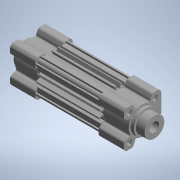
# Autodesk Inventor part: CP96S32-50(0)_BODY
Saved by Autodesk Inventor 2021 (Build 250183000, 183)
## iProperties
Part Number: CP96S32-50(0)_BODY
Material: Generic
Catalog Web Link: www.cadenas.de
Description: CP96 BODY-ISO Cylinder:Standard Double Acting,Single/Double Rod
Vendor: SMC
Document SubType Name: Modeling
Designer: partserver
Manufacturer: SMC
Mass: 188.486 g
Surface Area: 568.726 cm^2
Volume: 188.486 cm^3
Density: 1 g/cm^3
Appearance: PSOLRGB-192-192-192
Category: PARTsolutions
Company: SMC
PSOL_IDENT_0: {$CADENAS_DATA\23d-libs\smc_jp\actuator\standard_air_cylinder\cp96_c96\cp96\parts\cp96_body.prj},199
PSOL_IDENT_1: {VTYP=3D},{NB=CP96S32-50(0)_BODY},{LINA=CP96S32-50_BODY},{NN=CP96 BODY},{DATE=05.07.2021 01:48:16},
PSOL_IDENT_2: {GEOMDATE=28.11.2018 06:56:23},{VERSION=},{LINEID=10},{WBVAR=STROKE,ROD,THREAD},{WBNUMERIC=STROKE}
PSOL_IDENT_3: {NB=CP96S32-50(0)_BODY},{LINA=CP96S32-50_BODY},{KT=DUMMY},{BORE=32},{STROKE=50},{ROD=},{THREAD=0},{O
PSOL_IDENT_4: RDER=CP96S32-50},{A=22},{B=30},{D=12},{EE=G 1/8},{EEE=NPT 1/8},{EEND=9.728},{EED=9},{PL=13.0},{RT=M6
PSOL_IDENT_5: x1},{RTRA=6},{RTRP=1.00},{L12=6.0},{KK=M10x1.25},{SW=10},{G=32.0},{BG=16},{L8=94},{VD=4},{VA=4},{WA=
PSOL_IDENT_6: 4.0},{WB=7.0},{WH=26},{ZZ=146},{ZY=190},{E=47},{R=32.5},{L2=15},{L9=4},{H=48},{LC1=4.5},{LC2=25.5},{
PSOL_IDENT_7: RC1=1.5},{RC2=3.0},{RC3=6.8},{RC4=8.2},{RC5=3.9},{DC1=35.0},{DC2=36.0},{DC4=25.0},{HC=6.0},{C1=46.0}
PSOL_IDENT_8: ,{C2=42.0},{C3=30.5},{C4=34.5},{C5=16.5},{C6=20.5},{C7=17.8},{C9=17.5},{FONT=5},{SIZE=10}
NB: CP96S32-50(0)_BODY
NN: CP96 BODY
NT: ISO Cylinder:Standard Double Acting,Single/Double Rod
NBSYN: $ORDER.($THREAD.)_BODY
LINA: CP96S32-50_BODY
CATALOG: SMC (JP
BORE: 32
STROKE: 50
ROD: (-) Single rod
THREAD: on
A: 22
B: 30
D: 12
EE: G 1/8
EEE: NPT 1/8
PL: 13
RT: M6x1
L12: 6
KK: M10x1.25
SW: 10
G: 32
BG: 16
L8: 94
VD: 4
VA: 4
WA: 4
WB: 7
WH: 26
ZZ: 146
ZY: 190
E: 47
R: 32.5
L2: 15
L9: 4
H: 48
SUPPLIER: SMC
ARTICLENO: CP96S32-50(0)_BODY
BOMINFO: CP96S32-50_BODY
CREATOR: CADENAS GmbH
Title: CP96S32-50_BODY
Author: Cadenas PARTsolutions
Comments: ISO Cylinder:Standard Double Acting,Single/Double Rod
Autodesk Inventor part; units mm, degrees
sketch "Sketch_5" plane through (0, 0, 0) normal (1, 0, 0) x (0, 1, 0)
  line L0 (19.2462, 23.5) -> (14.2154, 23.5)
  arc A0 (14.2154, 23.5) -> (11.5708, 21.9163) centre (14.2154, 20.5) ccw
  line L1 (11.5708, 21.9163) -> (10.2555, 19.4602)
  arc A1 (10.2555, 19.4602) -> (9.4976, 17.0528) centre (16.25, 16.25) ccw
  arc A2 (7.3758, 15.8697) -> (9.4976, 17.0528) centre (8.0081, 17.2299) ccw
  arc A3 (7.3758, 15.8697) -> (-7.3758, 15.8697) centre (0, 0) ccw
  arc A4 (-9.4976, 17.0528) -> (-7.3758, 15.8697) centre (-8.0081, 17.2299) ccw
  arc A5 (-9.4976, 17.0528) -> (-10.2555, 19.4602) centre (-16.25, 16.25) ccw
  line L2 (-10.2555, 19.4602) -> (-11.5708, 21.9163)
  arc A6 (-11.5708, 21.9163) -> (-14.2154, 23.5) centre (-14.2154, 20.5) ccw
  line L3 (-14.2154, 23.5) -> (-19.2462, 23.5)
  arc A7 (-19.2462, 23.5) -> (-20.9749, 22.9519) centre (-19.2462, 20.5) ccw
  arc A8 (-20.9749, 22.9519) -> (-22.9519, 20.9749) centre (-16.25, 16.25) ccw
  arc A9 (-22.9519, 20.9749) -> (-23.5, 19.2462) centre (-20.5, 19.2462) ccw
  line L4 (-23.5, 19.2462) -> (-23.5, 14.2154)
  arc A10 (-23.5, 14.2154) -> (-21.9163, 11.5708) centre (-20.5, 14.2154) ccw
  line L5 (-21.9163, 11.5708) -> (-19.4602, 10.2555)
  arc A11 (-19.4602, 10.2555) -> (-17.0528, 9.4976) centre (-16.25, 16.25) ccw
  arc A12 (-15.8697, 7.3758) -> (-17.0528, 9.4976) centre (-17.2299, 8.0081) ccw
  arc A13 (-15.8697, 7.3758) -> (-15.8697, -7.3758) centre (0, 0) ccw
  arc A14 (-17.0528, -9.4976) -> (-15.8697, -7.3758) centre (-17.2299, -8.0081) ccw
  arc A15 (-17.0528, -9.4976) -> (-19.4602, -10.2555) centre (-16.25, -16.25) ccw
  line L6 (-19.4602, -10.2555) -> (-21.9163, -11.5708)
  arc A16 (-21.9163, -11.5708) -> (-23.5, -14.2154) centre (-20.5, -14.2154) ccw
  line L7 (-23.5, -14.2154) -> (-23.5, -19.2462)
  arc A17 (-23.5, -19.2462) -> (-22.9519, -20.9749) centre (-20.5, -19.2462) ccw
  arc A18 (-22.9519, -20.9749) -> (-20.9749, -22.9519) centre (-16.25, -16.25) ccw
  arc A19 (-20.9749, -22.9519) -> (-19.2462, -23.5) centre (-19.2462, -20.5) ccw
  line L8 (-19.2462, -23.5) -> (-14.2154, -23.5)
  arc A20 (-14.2154, -23.5) -> (-11.5708, -21.9163) centre (-14.2154, -20.5) ccw
  line L9 (-11.5708, -21.9163) -> (-10.2555, -19.4602)
  arc A21 (-10.2555, -19.4602) -> (-9.4976, -17.0528) centre (-16.25, -16.25) ccw
  arc A22 (-7.3758, -15.8697) -> (-9.4976, -17.0528) centre (-8.0081, -17.2299) ccw
  arc A23 (-7.3758, -15.8697) -> (7.3758, -15.8697) centre (0, 0) ccw
  arc A24 (9.4976, -17.0528) -> (7.3758, -15.8697) centre (8.0081, -17.2299) ccw
  arc A25 (9.4976, -17.0528) -> (10.2555, -19.4602) centre (16.25, -16.25) ccw
  line L10 (10.2555, -19.4602) -> (11.5708, -21.9163)
  arc A26 (11.5708, -21.9163) -> (14.2154, -23.5) centre (14.2154, -20.5) ccw
  line L11 (14.2154, -23.5) -> (19.2462, -23.5)
  arc A27 (19.2462, -23.5) -> (20.9749, -22.9519) centre (19.2462, -20.5) ccw
  arc A28 (20.9749, -22.9519) -> (22.9519, -20.9749) centre (16.25, -16.25) ccw
  arc A29 (22.9519, -20.9749) -> (23.5, -19.2462) centre (20.5, -19.2462) ccw
  line L12 (23.5, -19.2462) -> (23.5, -14.2154)
  arc A30 (23.5, -14.2154) -> (21.9163, -11.5708) centre (20.5, -14.2154) ccw
  line L13 (21.9163, -11.5708) -> (19.4602, -10.2555)
  arc A31 (19.4602, -10.2555) -> (17.0528, -9.4976) centre (16.25, -16.25) ccw
  arc A32 (15.8697, -7.3758) -> (17.0528, -9.4976) centre (17.2299, -8.0081) ccw
  arc A33 (15.8697, -7.3758) -> (15.8697, 7.3758) centre (0, 0) ccw
  arc A34 (17.0528, 9.4976) -> (15.8697, 7.3758) centre (17.2299, 8.0081) ccw
  arc A35 (17.0528, 9.4976) -> (19.4602, 10.2555) centre (16.25, 16.25) ccw
  line L14 (19.4602, 10.2555) -> (21.9163, 11.5708)
  arc A36 (21.9163, 11.5708) -> (23.5, 14.2154) centre (20.5, 14.2154) ccw
  line L15 (23.5, 14.2154) -> (23.5, 19.2462)
  arc A37 (23.5, 19.2462) -> (22.9519, 20.9749) centre (20.5, 19.2462) ccw
  arc A38 (22.9519, 20.9749) -> (20.9749, 22.9519) centre (16.25, 16.25) ccw
  arc A39 (20.9749, 22.9519) -> (19.2462, 23.5) centre (19.2462, 20.5) ccw
  constraints: 80 point on circle, 40 centre point, 32 end point
extrude "Extrusion1" add sketch "Sketch_5" along normal blind 32
sketch "Sketch_29" plane through (32, 0, 0) normal (1, 0, 0) x (0, 0, -1)
  line L0 (-23.0894, 1.6246) -> (-17.5, -0.031)
  arc A0 (-17.5, -0.031) -> (-17.3057, -2.6003) centre (0, 0) ccw
  line L1 (-17.3057, -2.6003) -> (-22.1807, -4.4229)
  line L2 (-22.1807, -4.4229) -> (-21.4365, -6.4134)
  line L3 (-21.4365, -6.4134) -> (-20.5984, -6.1)
  arc A1 (-19.5478, -8.91) -> (-20.5984, -6.1) centre (-18.6632, -6.9779) ccw
  line L4 (-19.5478, -8.91) -> (-21, -9.453)
  line L5 (-21, -9.453) -> (-21, -15.25)
  line L6 (-21, -15.25) -> (-23, -15.25)
  line L7 (-23, -15.25) -> (-23, -17.25)
  line L8 (-23, -17.25) -> (-21, -17.25)
  arc A2 (-21, -17.25) -> (-17.25, -21) centre (-17.25, -17.25) ccw
  line L9 (-17.25, -21) -> (-17.25, -23)
  line L10 (-17.25, -23) -> (-15.25, -23)
  line L11 (-15.25, -23) -> (-15.25, -21)
  line L12 (-15.25, -21) -> (-8.9843, -21)
  line L13 (-8.9843, -21) -> (-8.5904, -19.6702)
  line L14 (-8.5904, -19.6702) -> (-9.2136, -19.4856)
  line L15 (-9.2136, -19.4856) -> (-8.2196, -16.1297)
  line L16 (-8.2196, -16.1297) -> (-1.8914, -18.0042)
  line L17 (-1.8914, -18.0042) -> (-2.8854, -21.3601)
  line L18 (-2.8854, -21.3601) -> (-3.5087, -21.1755)
  line L19 (-3.5087, -21.1755) -> (-3.8779, -22.422)
  line L20 (-3.8779, -22.422) -> (-1.6246, -23.0894)
  line L21 (-1.6246, -23.0894) -> (0.031, -17.5)
  arc A3 (0.031, -17.5) -> (2.6003, -17.3057) centre (0, 0) ccw
  line L22 (2.6003, -17.3057) -> (4.4229, -22.1807)
  line L23 (4.4229, -22.1807) -> (6.4134, -21.4365)
  line L24 (6.4134, -21.4365) -> (6.1, -20.5984)
  arc A4 (8.91, -19.5478) -> (6.1, -20.5984) centre (6.9779, -18.6632) ccw
  line L25 (8.91, -19.5478) -> (9.453, -21)
  line L26 (9.453, -21) -> (15.25, -21)
  line L27 (15.25, -21) -> (15.25, -23)
  line L28 (15.25, -23) -> (17.25, -23)
  line L29 (17.25, -23) -> (17.25, -21)
  arc A5 (17.25, -21) -> (21, -17.25) centre (17.25, -17.25) ccw
  line L30 (21, -17.25) -> (23, -17.25)
  line L31 (23, -17.25) -> (23, -15.25)
  line L32 (23, -15.25) -> (21, -15.25)
  line L33 (21, -15.25) -> (21, -8.9843)
  line L34 (21, -8.9843) -> (19.6702, -8.5904)
  line L35 (19.6702, -8.5904) -> (19.4856, -9.2136)
  line L36 (19.4856, -9.2136) -> (16.1297, -8.2196)
  line L37 (16.1297, -8.2196) -> (18.0042, -1.8914)
  line L38 (18.0042, -1.8914) -> (21.3601, -2.8854)
  line L39 (21.3601, -2.8854) -> (21.1755, -3.5087)
  line L40 (21.1755, -3.5087) -> (22.422, -3.8779)
  line L41 (22.422, -3.8779) -> (23.0894, -1.6246)
  line L42 (23.0894, -1.6246) -> (17.5, 0.031)
  arc A6 (17.5, 0.031) -> (17.3057, 2.6003) centre (0, 0) ccw
  line L43 (17.3057, 2.6003) -> (22.1807, 4.4229)
  line L44 (22.1807, 4.4229) -> (21.4365, 6.4134)
  line L45 (21.4365, 6.4134) -> (20.5984, 6.1)
  arc A7 (19.5478, 8.91) -> (20.5984, 6.1) centre (18.6632, 6.9779) ccw
  line L46 (19.5478, 8.91) -> (21, 9.453)
  line L47 (21, 9.453) -> (21, 15.25)
  line L48 (21, 15.25) -> (23, 15.25)
  line L49 (23, 15.25) -> (23, 17.25)
  line L50 (23, 17.25) -> (21, 17.25)
  arc A8 (21, 17.25) -> (17.25, 21) centre (17.25, 17.25) ccw
  line L51 (17.25, 21) -> (17.25, 23)
  line L52 (17.25, 23) -> (15.25, 23)
  line L53 (15.25, 23) -> (15.25, 21)
  line L54 (15.25, 21) -> (8.9843, 21)
  line L55 (8.9843, 21) -> (8.5904, 19.6702)
  line L56 (8.5904, 19.6702) -> (9.2136, 19.4856)
  line L57 (9.2136, 19.4856) -> (8.2196, 16.1297)
  line L58 (8.2196, 16.1297) -> (1.8914, 18.0042)
  line L59 (1.8914, 18.0042) -> (2.8854, 21.3601)
  line L60 (2.8854, 21.3601) -> (3.5087, 21.1755)
  line L61 (3.5087, 21.1755) -> (3.8779, 22.422)
  line L62 (3.8779, 22.422) -> (1.6246, 23.0894)
  line L63 (1.6246, 23.0894) -> (-0.031, 17.5)
  arc A9 (-0.031, 17.5) -> (-2.6003, 17.3057) centre (0, 0) ccw
  line L64 (-2.6003, 17.3057) -> (-4.4229, 22.1807)
  line L65 (-4.4229, 22.1807) -> (-6.4134, 21.4365)
  line L66 (-6.4134, 21.4365) -> (-6.1, 20.5984)
  arc A10 (-8.91, 19.5478) -> (-6.1, 20.5984) centre (-6.9779, 18.6632) ccw
  line L67 (-8.91, 19.5478) -> (-9.453, 21)
  line L68 (-9.453, 21) -> (-15.25, 21)
  line L69 (-15.25, 21) -> (-15.25, 23)
  line L70 (-15.25, 23) -> (-17.25, 23)
  line L71 (-17.25, 23) -> (-17.25, 21)
  arc A11 (-17.25, 21) -> (-21, 17.25) centre (-17.25, 17.25) ccw
  line L72 (-21, 17.25) -> (-23, 17.25)
  line L73 (-23, 17.25) -> (-23, 15.25)
  line L74 (-23, 15.25) -> (-21, 15.25)
  line L75 (-21, 15.25) -> (-21, 8.9843)
  line L76 (-21, 8.9843) -> (-19.6702, 8.5904)
  line L77 (-19.6702, 8.5904) -> (-19.4856, 9.2136)
  line L78 (-19.4856, 9.2136) -> (-16.1297, 8.2196)
  line L79 (-16.1297, 8.2196) -> (-18.0042, 1.8914)
  line L80 (-18.0042, 1.8914) -> (-21.3601, 2.8854)
  line L81 (-21.3601, 2.8854) -> (-21.1755, 3.5087)
  line L82 (-21.1755, 3.5087) -> (-22.422, 3.8779)
  line L83 (-22.422, 3.8779) -> (-23.0894, 1.6246)
  constraints: 168 end point, 24 point on circle, 12 centre point
extrude "Extrusion2" add sketch "Sketch_29" along normal blind 80
sketch "Sketch_36" plane through (0, 23.5, 0) normal (0, 1, 0) x (1, 0, 0)
  line L0 (0, -4.5) -> (18, -4.5)
  arc A0 (18, -4.5) -> (21.5, -1) centre (18, -1) ccw
  arc A1 (22.5, 0) -> (21.5, -1) centre (22.5, -1) ccw
  line L1 (22.5, 0) -> (32, 0)
  line L2 (32, 0) -> (32, 16.25)
  line L3 (32, 16.25) -> (0, 16.25)
  line L4 (0, 16.25) -> (0, -4.5)
  constraints: 10 end point, 4 point on circle, 2 centre point
extrude "Extrusion3" add sketch "Sketch_36" against normal blind 12.25
sketch "Sketch_35" plane through (144, 0, 0) normal (1, 0, 0) x (0, 0, -1)
  line L0 (-23.5, 19.2462) -> (-23.5, 14.2154)
  arc A0 (-23.5, 14.2154) -> (-21.9163, 11.5708) centre (-20.5, 14.2154) ccw
  line L1 (-21.9163, 11.5708) -> (-19.4602, 10.2555)
  arc A1 (-19.4602, 10.2555) -> (-17.0528, 9.4976) centre (-16.25, 16.25) ccw
  arc A2 (-15.8697, 7.3758) -> (-17.0528, 9.4976) centre (-17.2299, 8.0081) ccw
  arc A3 (-15.8697, 7.3758) -> (-15.8697, -7.3758) centre (0, 0) ccw
  arc A4 (-17.0528, -9.4976) -> (-15.8697, -7.3758) centre (-17.2299, -8.0081) ccw
  arc A5 (-17.0528, -9.4976) -> (-19.4602, -10.2555) centre (-16.25, -16.25) ccw
  line L2 (-19.4602, -10.2555) -> (-21.9163, -11.5708)
  arc A6 (-21.9163, -11.5708) -> (-23.5, -14.2154) centre (-20.5, -14.2154) ccw
  line L3 (-23.5, -14.2154) -> (-23.5, -19.2462)
  arc A7 (-23.5, -19.2462) -> (-22.9519, -20.9749) centre (-20.5, -19.2462) ccw
  arc A8 (-22.9519, -20.9749) -> (-20.9749, -22.9519) centre (-16.25, -16.25) ccw
  arc A9 (-20.9749, -22.9519) -> (-19.2462, -23.5) centre (-19.2462, -20.5) ccw
  line L4 (-19.2462, -23.5) -> (-14.2154, -23.5)
  arc A10 (-14.2154, -23.5) -> (-11.5708, -21.9163) centre (-14.2154, -20.5) ccw
  line L5 (-11.5708, -21.9163) -> (-10.2555, -19.4602)
  arc A11 (-10.2555, -19.4602) -> (-9.4976, -17.0528) centre (-16.25, -16.25) ccw
  arc A12 (-7.3758, -15.8697) -> (-9.4976, -17.0528) centre (-8.0081, -17.2299) ccw
  arc A13 (-7.3758, -15.8697) -> (7.3758, -15.8697) centre (0, 0) ccw
  arc A14 (9.4976, -17.0528) -> (7.3758, -15.8697) centre (8.0081, -17.2299) ccw
  arc A15 (9.4976, -17.0528) -> (10.2555, -19.4602) centre (16.25, -16.25) ccw
  line L6 (10.2555, -19.4602) -> (11.5708, -21.9163)
  arc A16 (11.5708, -21.9163) -> (14.2154, -23.5) centre (14.2154, -20.5) ccw
  line L7 (14.2154, -23.5) -> (19.2462, -23.5)
  arc A17 (19.2462, -23.5) -> (20.9749, -22.9519) centre (19.2462, -20.5) ccw
  arc A18 (20.9749, -22.9519) -> (22.9519, -20.9749) centre (16.25, -16.25) ccw
  arc A19 (22.9519, -20.9749) -> (23.5, -19.2462) centre (20.5, -19.2462) ccw
  line L8 (23.5, -19.2462) -> (23.5, -14.2154)
  arc A20 (23.5, -14.2154) -> (21.9163, -11.5708) centre (20.5, -14.2154) ccw
  line L9 (21.9163, -11.5708) -> (19.4602, -10.2555)
  arc A21 (19.4602, -10.2555) -> (17.0528, -9.4976) centre (16.25, -16.25) ccw
  arc A22 (15.8697, -7.3758) -> (17.0528, -9.4976) centre (17.2299, -8.0081) ccw
  arc A23 (15.8697, -7.3758) -> (15.8697, 7.3758) centre (0, 0) ccw
  arc A24 (17.0528, 9.4976) -> (15.8697, 7.3758) centre (17.2299, 8.0081) ccw
  arc A25 (17.0528, 9.4976) -> (19.4602, 10.2555) centre (16.25, 16.25) ccw
  line L10 (19.4602, 10.2555) -> (21.9163, 11.5708)
  arc A26 (21.9163, 11.5708) -> (23.5, 14.2154) centre (20.5, 14.2154) ccw
  line L11 (23.5, 14.2154) -> (23.5, 19.2462)
  arc A27 (23.5, 19.2462) -> (22.9519, 20.9749) centre (20.5, 19.2462) ccw
  arc A28 (22.9519, 20.9749) -> (20.9749, 22.9519) centre (16.25, 16.25) ccw
  arc A29 (20.9749, 22.9519) -> (19.2462, 23.5) centre (19.2462, 20.5) ccw
  line L12 (19.2462, 23.5) -> (14.2154, 23.5)
  arc A30 (14.2154, 23.5) -> (11.5708, 21.9163) centre (14.2154, 20.5) ccw
  line L13 (11.5708, 21.9163) -> (10.2555, 19.4602)
  arc A31 (10.2555, 19.4602) -> (9.4976, 17.0528) centre (16.25, 16.25) ccw
  arc A32 (7.3758, 15.8697) -> (9.4976, 17.0528) centre (8.0081, 17.2299) ccw
  arc A33 (7.3758, 15.8697) -> (-7.3758, 15.8697) centre (0, 0) ccw
  arc A34 (-9.4976, 17.0528) -> (-7.3758, 15.8697) centre (-8.0081, 17.2299) ccw
  arc A35 (-9.4976, 17.0528) -> (-10.2555, 19.4602) centre (-16.25, 16.25) ccw
  line L14 (-10.2555, 19.4602) -> (-11.5708, 21.9163)
  arc A36 (-11.5708, 21.9163) -> (-14.2154, 23.5) centre (-14.2154, 20.5) ccw
  line L15 (-14.2154, 23.5) -> (-19.2462, 23.5)
  arc A37 (-19.2462, 23.5) -> (-20.9749, 22.9519) centre (-19.2462, 20.5) ccw
  arc A38 (-20.9749, 22.9519) -> (-22.9519, 20.9749) centre (-16.25, 16.25) ccw
  arc A39 (-22.9519, 20.9749) -> (-23.5, 19.2462) centre (-20.5, 19.2462) ccw
  constraints: 80 point on circle, 40 centre point, 32 end point
extrude "Extrusion4" add sketch "Sketch_35" against normal blind 32
sketch "Sketch_38" plane through (0, 23.5, 0) normal (0, 1, 0) x (1, 0, 0)
  line L0 (112, 0) -> (112, -16.25)
  line L1 (112, -16.25) -> (144, -16.25)
  line L2 (144, -16.25) -> (144, 4.5)
  line L3 (144, 4.5) -> (126, 4.5)
  arc A0 (126, 4.5) -> (122.5, 1) centre (126, 1) ccw
  arc A1 (121.5, 0) -> (122.5, 1) centre (121.5, 1) ccw
  line L4 (121.5, 0) -> (112, 0)
  constraints: 10 end point, 4 point on circle, 2 centre point
extrude "Extrusion5" add sketch "Sketch_38" against normal blind 12.25
sketch "Sketch_1" plane through (0, 0, 0) normal (0, 0, 1) x (1, 0, 0)
  line L0 (0, 0) -> (-15, 0)
  line L1 (-15, 0) -> (-15, 12.5)
  line L2 (-15, 12.5) -> (-4, 12.5)
  line L3 (-4, 12.5) -> (-4, 15)
  line L4 (-4, 15) -> (0, 15)
  line L5 (0, 15) -> (0, 0)
  line L6 (0, 0) -> (-15, 0)
  constraints: 14 end point
revolve "Revolution1" add sketch "Sketch_1" angle 360 about axis through (0, 0, 0) along (1, 0, 0)
sketch "Sketch_2" plane through (0, 0, 0) normal (0, 0, 1) x (1, 0, 0)
  line L0 (148, 0) -> (144, 0)
  line L1 (144, 0) -> (144, 15)
  line L2 (144, 15) -> (148, 15)
  line L3 (148, 15) -> (148, 0)
  line L4 (148, 0) -> (144, 0)
  constraints: 10 end point
revolve "Revolution2" add sketch "Sketch_2" angle 360 about axis through (148, 0, 0) along (1, 0, 0)
sketch "Sketch_3" plane through (0, 0, 0) normal (0, 0, 1) x (1, 0, 0)
  line L0 (92, 0) -> (-15, 0)
  line L1 (-15, 0) -> (-15, 6)
  line L2 (-15, 6) -> (32, 6)
  line L3 (32, 6) -> (32, 16)
  line L4 (32, 16) -> (92, 16)
  line L5 (92, 16) -> (92, 0)
  line L6 (92, 0) -> (-15, 0)
  constraints: 14 end point
revolve "Revolution3" cut sketch "Sketch_3" angle 360 about axis through (92, 0, 0) along (1, 0, 0)
sketch "Sketch_25" plane through (0, 0, -16.25) normal (0, 0, 1) x (1, 0, 0)
  line L0 (17.4194, 16.25) -> (0, 16.25)
  line L1 (0, 16.25) -> (0, 18.25)
  line L2 (0, 18.25) -> (4, 18.25)
  line L3 (4, 18.25) -> (4, 19.25)
  line L4 (4, 19.25) -> (4.5415, 18.7085)
  line L5 (4.5415, 18.7085) -> (16, 18.7085)
  line L6 (16, 18.7085) -> (17.4194, 16.25)
  line L7 (17.4194, 16.25) -> (0, 16.25)
  constraints: 16 end point
revolve "Revolution4" cut sketch "Sketch_25" angle 360 about axis through (17.4194, 16.25, -16.25) along (1, 0, 0)
thread "Thread1" size "M6x1" class "6H" standard "ISO Metric profile" full length
pattern_linear "Rectangular Pattern1" count 2 spacing 32.5 along (0, 0, 1) count 2 spacing 32.5 along (0, -1, 0) of "Revolution4"
sketch "Sketch_6" plane through (0, 0, 0) normal (1, 0, 0) x (0, 1, 0)
  line L0 (14.5179, -13.25) -> (12.7859, -16.25)
  line L1 (12.7859, -16.25) -> (14.5179, -19.25)
  line L2 (14.5179, -19.25) -> (17.9821, -19.25)
  line L3 (17.9821, -19.25) -> (19.7141, -16.25)
  line L4 (19.7141, -16.25) -> (17.9821, -13.25)
  line L5 (17.9821, -13.25) -> (14.5179, -13.25)
  constraints: 12 end point
extrude "Extrusion6" cut sketch "Sketch_6" along normal blind 4
pattern_linear "Rectangular Pattern2" count 2 spacing 32.5 along (0, 0, 1) count 2 spacing 32.5 along (0, -1, 0) of "Extrusion6"
sketch "Sketch_26" plane through (0, 0, -16.25) normal (0, 0, 1) x (1, 0, 0)
  line L0 (144, 16.25) -> (126.5806, 16.25)
  line L1 (126.5806, 16.25) -> (128, 18.7085)
  line L2 (128, 18.7085) -> (139.4585, 18.7085)
  line L3 (139.4585, 18.7085) -> (140, 19.25)
  line L4 (140, 19.25) -> (140, 18.25)
  line L5 (140, 18.25) -> (144, 18.25)
  line L6 (144, 18.25) -> (144, 16.25)
  line L7 (144, 16.25) -> (126.5806, 16.25)
  constraints: 16 end point
revolve "Revolution5" cut sketch "Sketch_26" angle 360 about axis through (144, 16.25, -16.25) along (1, 0, 0)
thread "Thread2" size "M6x1" class "6H" standard "ISO Metric profile" full length
pattern_linear "Rectangular Pattern3" count 2 spacing 32.5 along (0, 0, 1) count 2 spacing 32.5 along (0, -1, 0) of "Revolution5"
sketch "Sketch_12" plane through (144, 0, 0) normal (1, 0, 0) x (0, 0, -1)
  line L0 (13.25, 14.5179) -> (16.25, 12.7859)
  line L1 (16.25, 12.7859) -> (19.25, 14.5179)
  line L2 (19.25, 14.5179) -> (19.25, 17.9821)
  line L3 (19.25, 17.9821) -> (16.25, 19.7141)
  line L4 (16.25, 19.7141) -> (13.25, 17.9821)
  line L5 (13.25, 17.9821) -> (13.25, 14.5179)
  constraints: 12 end point
extrude "Extrusion7" cut sketch "Sketch_12" against normal blind 4
pattern_linear "Rectangular Pattern4" count 2 spacing 32.5 along (0, 0, 1) count 2 spacing 32.5 along (0, -1, 0) of "Extrusion7"
sketch "Sketch_20" plane through (13, 0, 0) normal (1, 0, 0) x (0, 0, -1)
  line L0 (4, 12.0272) -> (4, 23.5)
  line L1 (4, 23.5) -> (8.864, 23.5)
  line L2 (8.864, 23.5) -> (8.283, 22.919)
  line L3 (8.283, 22.919) -> (8.283, 14.5)
  line L4 (8.283, 14.5) -> (4, 12.0272)
  line L5 (4, 12.0272) -> (4, 23.5)
  constraints: 12 end point
revolve "Revolution6" cut sketch "Sketch_20" angle 360 about axis through (13, 12.0272, -4) along (0, -1, 0)
thread "Thread3" size "G9.728x0.907" designation "G 1/8" standard "ISO Pipe Threads" full length
sketch "Sketch_21" plane through (0, 0, -7) normal (0, 0, 1) x (1, 0, 0)
  line L0 (25.5, 18.5) -> (25.5, 23.5)
  line L1 (25.5, 23.5) -> (29.4, 23.5)
  line L2 (29.4, 23.5) -> (29.4, 18.5)
  line L3 (29.4, 18.5) -> (25.5, 18.5)
  line L4 (25.5, 18.5) -> (25.5, 23.5)
  constraints: 10 end point
revolve "Revolution7" cut sketch "Sketch_21" angle 360 about axis through (25.5, 18.5, -7) along (0, -1, 0)
sketch "Sketch_23" plane through (131, 0, 0) normal (1, 0, 0) x (0, 0, -1)
  line L0 (-4, 12.0272) -> (-4, 23.5)
  line L1 (-4, 23.5) -> (0.864, 23.5)
  line L2 (0.864, 23.5) -> (0.283, 22.919)
  line L3 (0.283, 22.919) -> (0.283, 14.5)
  line L4 (0.283, 14.5) -> (-4, 12.0272)
  line L5 (-4, 12.0272) -> (-4, 23.5)
  constraints: 12 end point
revolve "Revolution8" cut sketch "Sketch_23" angle 360 about axis through (131, 12.0272, 4) along (0, -1, 0)
thread "Thread4" size "G9.728x0.907" designation "G 1/8" standard "ISO Pipe Threads" full length
sketch "Sketch_24" plane through (0, 0, 7) normal (0, 0, 1) x (1, 0, 0)
  line L0 (118.5, 18.5) -> (118.5, 23.5)
  line L1 (118.5, 23.5) -> (122.4, 23.5)
  line L2 (122.4, 23.5) -> (122.4, 18.5)
  line L3 (122.4, 18.5) -> (118.5, 18.5)
  line L4 (118.5, 18.5) -> (118.5, 23.5)
  constraints: 10 end point
revolve "Revolution9" cut sketch "Sketch_24" angle 360 about axis through (118.5, 18.5, 7) along (0, -1, 0)
ref_plane "BODY_BL_XY" through (0, 0, 0) normal (-1, 0, 0) x (0, 0, -1)
ref_plane "BODY_BL_YZ" through (0, 0, 0) normal (0, 0, -1) x (0, -1, 0)
ref_plane "BODY_BL_ZX" through (0, 0, 0) normal (0, -1, 0) x (-1, 0, 0)
ref_plane "BODY_BL1_XY" through (144, 0, 0) normal (1, 0, 0) x (0, 0, -1)
ref_plane "BODY_BL1_YZ" through (144, 0, 0) normal (0, 0, -1) x (0, 1, 0)
ref_plane "BODY_BL1_ZX" through (144, 0, 0) normal (0, 1, 0) x (1, 0, 0)
ref_plane "BODY_BR_XY" through (0, 0, 0) normal (-1, 0, 0) x (0, 0, -1)
ref_plane "BODY_BR_YZ" through (0, 0, 0) normal (0, 0, -1) x (0, -1, 0)
ref_plane "BODY_BR_ZX" through (0, 0, 0) normal (0, -1, 0) x (-1, 0, 0)
ref_plane "BODY_BR1_XY" through (144, 0, 0) normal (1, 0, 0) x (0, 0, -1)
ref_plane "BODY_BR1_YZ" through (144, 0, 0) normal (0, 0, -1) x (0, 1, 0)
ref_plane "BODY_BR1_ZX" through (144, 0, 0) normal (0, 1, 0) x (1, 0, 0)
ref_plane "BODY_DUMMY_XY" through (0, 0, 0) normal (-1, 0, 0) x (0, 0, -1)
ref_plane "BODY_DUMMY_YZ" through (0, 0, 0) normal (0, 0, -1) x (0, -1, 0)
ref_plane "BODY_DUMMY_ZX" through (0, 0, 0) normal (0, -1, 0) x (-1, 0, 0)
ref_plane "BODY_MOUNT1_XY" through (0, 0, 0) normal (-1, 0, 0) x (0, 0, -1)
ref_plane "BODY_MOUNT1_YZ" through (0, 0, 0) normal (0, 0, -1) x (0, -1, 0)
ref_plane "BODY_MOUNT1_ZX" through (0, 0, 0) normal (0, -1, 0) x (-1, 0, 0)
ref_plane "BODY_MOUNT2_XY" through (144, 0, 0) normal (1, 0, 0) x (0, 0, -1)
ref_plane "BODY_MOUNT2_YZ" through (144, 0, 0) normal (0, 0, -1) x (0, 1, 0)
ref_plane "BODY_MOUNT2_ZX" through (144, 0, 0) normal (0, 1, 0) x (1, 0, 0)
ref_plane "BODY_ROD_XY" through (0, 0, 0) normal (1, 0, 0) x (0, 0, -1)
ref_plane "BODY_ROD_YZ" through (0, 0, 0) normal (0, 0, -1) x (0, 1, 0)
ref_plane "BODY_ROD_ZX" through (0, 0, 0) normal (0, 1, 0) x (1, 0, 0)
ref_plane "BODY_SWA1_XY" through (32, 18.6632, 6.9779) normal (-1, 0, 0) x (0, 0.3502074, -0.9366722)
ref_plane "BODY_SWA1_YZ" through (32, 18.6632, 6.9779) normal (0, 0.3502074, -0.9366722) x (0, -0.9366722, -0.3502074)
ref_plane "BODY_SWA1_ZX" through (32, 18.6632, 6.9779) normal (0, -0.9366722, -0.3502074) x (-1, 0, 0)
ref_plane "BODY_SWB1_XY" through (112, -6.9779, 18.6632) normal (1, 0, 0) x (0, 0.3502074, -0.9366722)
ref_plane "BODY_SWB1_YZ" through (112, -6.9779, 18.6632) normal (0, 0.3502074, -0.9366722) x (0, 0.9366722, 0.3502074)
ref_plane "BODY_SWB1_ZX" through (112, -6.9779, 18.6632) normal (0, 0.9366722, 0.3502074) x (1, 0, 0)
ref_plane "G3_XY" through (112, 0, 0) normal (0, 1, 0) x (1, 0, 0)
ref_plane "G3_YZ" through (112, 0, 0) normal (1, 0, 0) x (0, 0, -1)
ref_plane "G3_ZX" through (112, 0, 0) normal (0, 0, -1) x (0, 1, 0)
ref_plane "G4_XY" through (144, 0, 0) normal (0, 1, 0) x (1, 0, 0)
ref_plane "G4_YZ" through (144, 0, 0) normal (1, 0, 0) x (0, 0, -1)
ref_plane "G4_ZX" through (144, 0, 0) normal (0, 0, -1) x (0, 1, 0)
ref_plane "R4_XY" through (0, 16.25, -16.25) normal (1, 0, 0) x (0, 0, -1)
ref_plane "R4_YZ" through (0, 16.25, -16.25) normal (0, 0, -1) x (0, 1, 0)
ref_plane "R4_ZX" through (0, 16.25, -16.25) normal (0, 1, 0) x (1, 0, 0)
ref_plane "VA2_XY" through (148, 0, 0) normal (0, 1, 0) x (1, 0, 0)
ref_plane "VA2_YZ" through (148, 0, 0) normal (1, 0, 0) x (0, 0, -1)
ref_plane "VA2_ZX" through (148, 0, 0) normal (0, 0, -1) x (0, 1, 0)
ref_plane "WA2_XY" through (13, 23.5, 0) normal (0, 1, 0) x (1, 0, 0)
ref_plane "WA2_YZ" through (13, 23.5, 0) normal (1, 0, 0) x (0, 0, -1)
ref_plane "WA2_ZX" through (13, 23.5, 0) normal (0, 0, -1) x (0, 1, 0)
body "Solid1"
